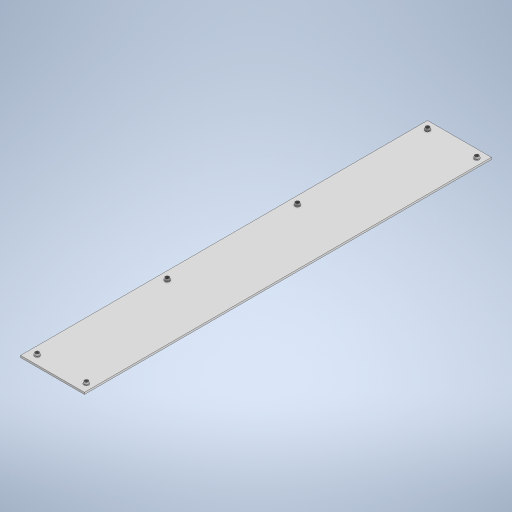
# Autodesk Inventor part: chapa_frente_esquerda
Saved by Autodesk Inventor 2024 (Build 280153000, 153)
## iProperties
Created: 2024-10-17
Part Number: chapa_frente_esquerda
Material: Genérico
Document SubType Name: Modeling
Designer: robof
Density: 1 g/cm^3
Appearance: Padrão
Author: robof
Autodesk Inventor part; units mm, degrees
ref_plane "YZ Plane" through (0, 0, 0) normal (1, 0, 0) x (0, 1, 0)
ref_plane "XZ Plane" through (0, 0, 0) normal (0, 1, 0) x (-1, 0, 0)
ref_plane "XY Plane" through (0, 0, 0) normal (0, 0, 1) x (1, 0, 0)
sketch "Esboço1" plane through (0, 0, 0) normal (0, 1, 0) x (-1, 0, 0)
  line L0 (0, 0) -> (-100.5, 0)
  line L1 (-100.5, 0) -> (-100.5, -640.37)
  line L2 (-100.5, -640.37) -> (0, -640.37)
  line L3 (0, -640.37) -> (0, 0)
  dimension "d0" = 100.5
  dimension "d1" = 640.37
  constraints: 8 end point, 2 parallel, 1 horizontal, 1 perpendicular
  measures "d0" distance of L2.end L1.end
  measures "d1" distance of L1.end L0.end
extrude "Extrusão1" add sketch "Esboço1" along normal blind 3
sketch "Esboço2" plane through (0, 3, 0) normal (0, 1, 0) x (1, 0, 0)
  line L0 (0, 0) -> (100.5, 0) projected
  line L1 (0, 0) -> (100.5, 0)
  line L2 (0, 20) -> (0, 0)
  line L3 (100.5, 640.37) -> (0, 640.37) projected
  line L4 (0, 0) -> (23, 0)
  line L5 (23, 0) -> (23, 640.37)
  line L6 (23, 640.37) -> (0, 640.37)
  line L7 (0, 640.37) -> (0, 0)
  line L8 (0, 640.37) -> (3, 640.37)
  line L9 (3, 640.37) -> (3, 0)
  line L10 (3, 0) -> (0, 0)
  line L11 (0, 0) -> (0, 640.37)
  line L12 (100.5, 0) -> (100.5, 640.37) projected
  line L13 (0, 0) -> (100.5, 0)
  line L14 (100.5, 0) -> (100.5, 23)
  line L15 (100.5, 23) -> (0, 23)
  line L16 (0, 23) -> (0, 0)
  line L17 (0, 23) -> (100.5, 23)
  line L18 (100.5, 23) -> (100.5, 3)
  line L19 (100.5, 3) -> (0, 3)
  line L20 (0, 3) -> (0, 23)
  line L21 (0, 640.37) -> (100.5, 640.37)
  line L22 (100.5, 640.37) -> (100.5, 617.37)
  line L23 (100.5, 617.37) -> (0, 617.37)
  line L24 (0, 617.37) -> (0, 640.37)
  line L25 (0, 617.37) -> (100.5, 617.37)
  line L26 (100.5, 617.37) -> (100.5, 637.37)
  line L27 (100.5, 637.37) -> (0, 637.37)
  line L28 (0, 637.37) -> (0, 617.37)
  line L29 (3, 617.37) -> (13, 617.37)
  line L30 (13, 617.37) -> (13, 627.37)
  line L31 (13, 627.37) -> (3, 627.37)
  line L32 (3, 627.37) -> (3, 617.37)
  line L33 (100.5, 617.37) -> (90.5, 617.37)
  line L34 (90.5, 617.37) -> (90.5, 627.37)
  line L35 (90.5, 627.37) -> (100.5, 627.37)
  line L36 (100.5, 627.37) -> (100.5, 617.37)
  line L37 (0, 320.185) -> (42.8938, 320.185)
  line L38 (0, 320.185) -> (13, 320.185)
  circle A0 centre (13, 320.185) radius 3
  circle A1 centre (13, 627.37) radius 3
  circle A2 centre (90.5, 627.37) radius 3
  line L39 (13, 320.185) -> (13, 422.58)
  line L40 (13, 422.58) -> (13, 524.975)
  circle A3 centre (13, 422.58) radius 3
  circle A4 centre (13, 524.975) radius 3
  circle A5 centre (13, 320.185) radius 3
  circle A6 centre (13, 13) radius 3
  circle A7 centre (90.5, 13) radius 3
  circle A8 centre (13, 217.79) radius 3
  circle A9 centre (13, 115.395) radius 3
  dimension "d5" = 23
  dimension "d6" = 3
  dimension "d7" = 23
  dimension "d8" = 20
  dimension "d9" = 23
  dimension "d10" = 20
  dimension "d11" = 10
  dimension "d12" = 10
  dimension "d13" = 10
  dimension "d14" = 6
  dimension "d15" = 6
  dimension "d16" = 6
  dimension "d17" = 102.395
  dimension "d18" = 102.395
  constraints: 76 end point, 16 parallel, 11 point on line, 10 centre point, 9 horizontal, 9 perpendicular, 5 coincident, 4 symmetric about line, 1 midpoint, 5 other
  measures "d5" distance of L6.end L5.end
  measures "d6" distance of L9.end L10.end
  measures "d7" distance of L14.end L13.end
  measures "d8" distance of L17.end L18.end
  measures "d9" distance of L21.end L22.end
  measures "d10" distance of L26.end L25.end
  measures "d11" distance of L31.end L30.end
  measures "d12" distance of L30.end L29.end
  measures "d13" distance of L34.end L35.end
  measures "d14" diameter of A0
  measures "d15" diameter of A1
  measures "d16" diameter of A2
  measures "d17" distance of L39.start L39.end
  measures "d18" distance of L39.end L40.end
extrude "Extrusão2" add sketch "Esboço2" along normal blind 4 contours A4 | A3 L40 L39 | L39 L40 A3 | A0 L39 L37 | L37 A0 | L37 L39 A0 | A1 L30 L31 | L31 L30 A1 | A2 L34 L35 | L35 L34 A2 | A6 | A7 | A8 | A9
sketch "Esboço3" plane through (0, 3, 0) normal (0, 1, 0) x (1, 0, 0)
  circle A0 centre (13, 13) radius 3 projected
  circle A1 centre (13, 13) radius 4
  circle A2 centre (90.5, 13) radius 3 projected
  circle A3 centre (90.5, 13) radius 4
  circle A4 centre (13, 115.395) radius 3 projected
  circle A5 centre (13, 115.395) radius 4
  circle A6 centre (13, 217.79) radius 3 projected
  circle A7 centre (13, 217.79) radius 4
  circle A8 centre (13, 320.185) radius 3 projected
  circle A9 centre (13, 320.185) radius 4
  line L0 (100.5, 0) -> (100.5, 640.37) projected
  line L1 (100.5, 320.185) -> (82.1081, 320.185)
  circle A10 centre (13, 627.37) radius 3
  circle A11 centre (13, 627.37) radius 4
  circle A12 centre (90.5, 627.37) radius 3
  circle A13 centre (90.5, 627.37) radius 4
  circle A14 centre (13, 524.975) radius 3
  circle A15 centre (13, 524.975) radius 4
  circle A16 centre (13, 422.58) radius 3
  circle A17 centre (13, 422.58) radius 4
  circle A18 centre (13, 320.185) radius 3
  circle A19 centre (13, 320.185) radius 4
  point P0 (0, 0)
  dimension "d21" = 8
  dimension "d22" = 8
  dimension "d23" = 8
  dimension "d24" = 8
  dimension "d25" = 8
  constraints: 15 centre point, 10 coincident, 8 symmetric about line, 2 end point, 1 horizontal, 1 midpoint, 10 other
  measures "d21" diameter of A1
  measures "d22" diameter of A3
  measures "d23" diameter of A5
  measures "d24" diameter of A7
  measures "d25" diameter of A9
extrude "Extrusão3" add sketch "Esboço3" along normal blind 1 contours A0 | A1 | A2 | A3 | A4 | A5 | A6 | A7 | A8 | A9 | A10 | A11 | A12 | A13 | A14 | A15 | A16 | A17
sketch "Esboço4" plane through (13, 7, -13) normal (0, 1, 0) x (1, 0, 0)
  circle A0 centre (0, 0) radius 3 projected
  line L0 (0, 0) -> (1.5, 0)
  circle A1 centre (0, 0) radius 4 projected
  line L1 (1.5, 0) -> (0.75, -1.299)
  line L2 (0.75, -1.299) -> (-0.75, -1.299)
  line L3 (-0.75, -1.299) -> (-1.5, 0)
  line L4 (-1.5, 0) -> (-0.75, 1.299)
  line L5 (-0.75, 1.299) -> (0.75, 1.299)
  line L6 (0.75, 1.299) -> (1.5, 0)
  circle A2 centre (77.5, 0) radius 3 projected
  line L7 (77.5, 0) -> (79, 0)
  line L8 (79, 0) -> (78.25, -1.299)
  line L9 (78.25, -1.299) -> (76.75, -1.299)
  line L10 (76.75, -1.299) -> (76, 0)
  line L11 (76, 0) -> (76.75, 1.299)
  line L12 (76.75, 1.299) -> (78.25, 1.299)
  line L13 (78.25, 1.299) -> (79, 0)
  circle A3 centre (0, 102.395) radius 3 projected
  line L14 (0, 102.395) -> (1.5, 102.395)
  line L15 (1.5, 102.395) -> (0.75, 101.096)
  line L16 (0.75, 101.096) -> (-0.75, 101.096)
  line L17 (-0.75, 101.096) -> (-1.5, 102.395)
  line L18 (-1.5, 102.395) -> (-0.75, 103.694)
  line L19 (-0.75, 103.694) -> (0.75, 103.694)
  line L20 (0.75, 103.694) -> (1.5, 102.395)
  circle A4 centre (0, 204.79) radius 3 projected
  line L21 (0, 204.79) -> (1.5, 204.79)
  line L22 (1.5, 204.79) -> (0.75, 203.491)
  line L23 (0.75, 203.491) -> (-0.75, 203.491)
  line L24 (-0.75, 203.491) -> (-1.5, 204.79)
  line L25 (-1.5, 204.79) -> (-0.75, 206.089)
  line L26 (-0.75, 206.089) -> (0.75, 206.089)
  line L27 (0.75, 206.089) -> (1.5, 204.79)
  circle A5 centre (0, 307.185) radius 4 projected
  line L28 (0, 307.185) -> (1.5, 307.185)
  circle A6 centre (0, 307.185) radius 3 projected
  line L29 (1.5, 307.185) -> (0.75, 305.886)
  line L30 (0.75, 305.886) -> (-0.75, 305.886)
  line L31 (-0.75, 305.886) -> (-1.5, 307.185)
  line L32 (-1.5, 307.185) -> (-0.75, 308.484)
  line L33 (-0.75, 308.484) -> (0.75, 308.484)
  line L34 (0.75, 308.484) -> (1.5, 307.185)
  line L35 (87.5, -13) -> (87.5, 627.37) projected
  line L36 (87.5, 307.185) -> (57.6178, 307.185)
  circle A7 centre (0, 614.37) radius 3
  line L37 (0, 614.37) -> (1.5, 614.37)
  circle A8 centre (0, 614.37) radius 4
  line L38 (1.5, 614.37) -> (0.75, 615.669)
  line L39 (0.75, 615.669) -> (-0.75, 615.669)
  line L40 (-0.75, 615.669) -> (-1.5, 614.37)
  line L41 (-1.5, 614.37) -> (-0.75, 613.071)
  line L42 (-0.75, 613.071) -> (0.75, 613.071)
  line L43 (0.75, 613.071) -> (1.5, 614.37)
  circle A9 centre (77.5, 614.37) radius 3
  line L44 (77.5, 614.37) -> (79, 614.37)
  line L45 (79, 614.37) -> (78.25, 615.669)
  line L46 (78.25, 615.669) -> (76.75, 615.669)
  line L47 (76.75, 615.669) -> (76, 614.37)
  line L48 (76, 614.37) -> (76.75, 613.071)
  line L49 (76.75, 613.071) -> (78.25, 613.071)
  line L50 (78.25, 613.071) -> (79, 614.37)
  circle A10 centre (0, 511.975) radius 3
  line L51 (0, 511.975) -> (1.5, 511.975)
  line L52 (1.5, 511.975) -> (0.75, 513.274)
  line L53 (0.75, 513.274) -> (-0.75, 513.274)
  line L54 (-0.75, 513.274) -> (-1.5, 511.975)
  line L55 (-1.5, 511.975) -> (-0.75, 510.676)
  line L56 (-0.75, 510.676) -> (0.75, 510.676)
  line L57 (0.75, 510.676) -> (1.5, 511.975)
  circle A11 centre (0, 409.58) radius 3
  line L58 (0, 409.58) -> (1.5, 409.58)
  line L59 (1.5, 409.58) -> (0.75, 410.879)
  line L60 (0.75, 410.879) -> (-0.75, 410.879)
  line L61 (-0.75, 410.879) -> (-1.5, 409.58)
  line L62 (-1.5, 409.58) -> (-0.75, 408.281)
  line L63 (-0.75, 408.281) -> (0.75, 408.281)
  line L64 (0.75, 408.281) -> (1.5, 409.58)
  circle A12 centre (0, 307.185) radius 4
  circle A13 centre (0, 307.185) radius 3
  line L65 (1.5, 307.185) -> (0.75, 308.484)
  line L66 (0.75, 308.484) -> (-0.75, 308.484)
  line L67 (-0.75, 308.484) -> (-1.5, 307.185)
  line L68 (-1.5, 307.185) -> (-0.75, 305.886)
  line L69 (-0.75, 305.886) -> (0.75, 305.886)
  line L70 (0.75, 305.886) -> (1.5, 307.185)
  point P0 (-13, -13)
  dimension "d28" = 1.5
  dimension "d29" = 1.5
  dimension "d30" = 1.5
  constraints: 140 end point, 37 symmetric about line, 10 coincident, 7 centre point, 6 horizontal, 1 midpoint, 72 other
  measures "d28" distance of L0.start L0.end
  measures "d29" distance of L7.start L7.end
  measures "d30" distance of L14.start L14.end
extrude "Extrusão4" cut sketch "Esboço4" against normal blind 1.5 contours L1 L2 L3 L4 L5 L6 | L8 L9 L10 L11 L12 L13 | L15 L16 L17 L18 L19 L20 | L22 L23 L24 L25 L26 L27 | L29 L30 L31 L32 L33 L34 | L43 L42 L41 L40 L39 L38 | L50 L49 L48 L47 L46 L45 | L57 L56 L55 L54 L53 L52 | L64 L63 L62 L61 L60 L59
sketch "Esboço5" plane through (0, 3, 0) normal (0, 1, 0) x (1, 0, 0)
  line L0 (4.5679, 103.4306) -> (23.4921, 103.4306)
  line L1 (23.4921, 103.4306) -> (23.4921, 130.838)
  line L2 (23.4921, 130.838) -> (4.5679, 130.838)
  line L3 (4.5679, 130.838) -> (4.5679, 103.4306)
  line L4 (4.5679, 310.9443) -> (23.4921, 310.9443)
  line L5 (23.4921, 310.9443) -> (23.4921, 337.6992)
  line L6 (23.4921, 337.6992) -> (4.5679, 337.6992)
  line L7 (4.5679, 337.6992) -> (4.5679, 310.9443)
  line L8 (4.5679, 512.5849) -> (23.4921, 512.5849)
  line L9 (23.4921, 512.5849) -> (23.4921, 537.3821)
  line L10 (23.4921, 537.3821) -> (4.5679, 537.3821)
  line L11 (4.5679, 537.3821) -> (4.5679, 512.5849)
  point P0 (0, 0)
  constraints: 24 end point, 6 parallel, 4 point on line, 3 horizontal, 3 perpendicular
extrude "Extrusão5" cut sketch "Esboço5" along normal blind 5
